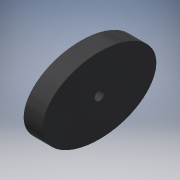
# Autodesk Inventor part: Cam
Saved by Autodesk Inventor 2016 (Build 200138000, 138)
## iProperties
Created: 2014-03-13
Part Number: Cam
Material: Rubber
Document SubType Name: Modeling
Designer: John
Density: 1 g/cm^3
Appearance: Rubber - Black - Version 1.1
Author: John
Autodesk Inventor part; units mm, degrees
ref_plane "YZ Plane" through (0, 0, 0) normal (1, 0, 0) x (0, 1, 0)
ref_plane "XZ Plane" through (0, 0, 0) normal (0, 1, 0) x (-1, 0, 0)
ref_plane "XY Plane" through (0, 0, 0) normal (0, 0, 1) x (1, 0, 0)
sketch "Sketch1" plane through (0, 0, 0) normal (1, 0, 0) x (0, 1, 0)
  ellipse E0 centre (0, 0) end of major axis (12.7, 0) minor radius 19.05
  dimension "d0" = 12.7
  dimension "d1" = 19.05
  constraints: 1 coincident, 2 other
extrude "Extrusion1" add sketch "Sketch1" along normal blind 6.35
sketch "Sketch2" plane through (6.35, 0, 0) normal (1, 0, 0) x (0, 0, -1)
  ellipse E0 centre (0, 0) end of major axis (-19.05, 0) minor radius 12.7 projected
  constraints: 1 other
hole "Hole1" at (6.35, 0, 0) direction (-1, 0, 0) diameter 3.175 end through all
body "Solid1"
